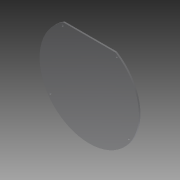
# Autodesk Inventor part: Top Plate
Saved by Autodesk Inventor 2015 (Build 190159000, 159)
## iProperties
Created: 2016-09-20
Part Number: Top Plate
Material: Generic
Document SubType Name: Modeling
Designer: James Yelland
Density: 1 g/cm^3
Appearance: Default
Author: James Yelland
Autodesk Inventor part; units mm, degrees
ref_plane "YZ Plane" through (0, 0, 0) normal (1, 0, 0) x (0, 1, 0)
ref_plane "XZ Plane" through (0, 0, 0) normal (0, 1, 0) x (-1, 0, 0)
ref_plane "XY Plane" through (0, 0, 0) normal (0, 0, 1) x (1, 0, 0)
sketch "Sketch1" plane through (0, 0, 0) normal (0, 1, 0) x (-1, 0, 0)
  circle A0 centre (-54.4898, 77.8194) radius 1.6
  circle A1 centre (54.4898, 77.8194) radius 1.6
  circle A2 centre (-78.9896, -52.7792) radius 1.6
  circle A3 centre (78.9896, -52.7792) radius 1.6
  line L0 (0, 85) -> (51.2348, 85)
  line L1 (0, 85) -> (-51.2348, 85)
  arc A4 (-53.9313, 84.2105) -> (53.9313, 84.2105) centre (0, 0) ccw
  arc A5 (53.9313, 84.2105) -> (51.2348, 85) centre (51.2348, 80) ccw
  arc A6 (-51.2348, 85) -> (-53.9313, 84.2105) centre (-51.2348, 80) ccw
  point P0 (-54.3117, 78)
  point P1 (54.3117, 78)
  point P2 (52.6783, 85)
  point P3 (-52.6783, 85)
  dimension "d11" = 3.2
  dimension "d12" = 3.2
  dimension "d13" = 3.2
  dimension "d14" = 3.2
  dimension "d20" = 5
  constraints: 8 point on circle, 7 centre point, 4 end point, 4 tangent, 3 point on line, 1 coincident, 1 equal radius, 1 horizontal
  measures "d11" diameter of A0
  measures "d12" diameter of A1
  measures "d13" diameter of A2
  measures "d14" diameter of A3
  measures "d20" radius of A5
extrude "Extrusion1" add sketch "Sketch1" along normal blind 3
body "Solid1"
